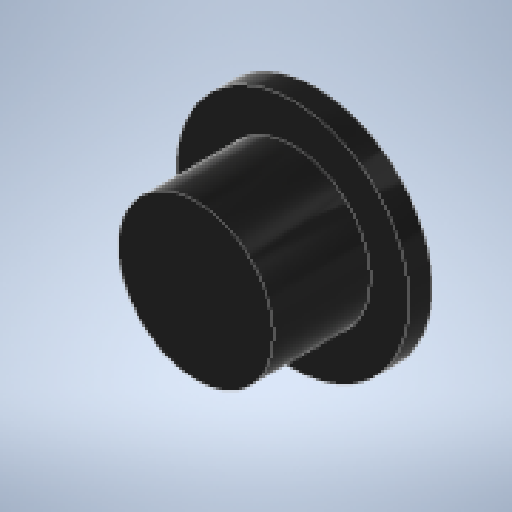
# Autodesk Inventor part: bouton
Saved by Autodesk Inventor 2024.2 (Build 282272000, 272)
## iProperties
Created: 2024-09-16
Part Number: bouton
Material: Plastique ABS
Document SubType Name: Modeling
Designer: Sebastien
Density: 1.06 g/cm^3
Appearance: Lisse - Noir
Author: Sebastien
Autodesk Inventor part; units mm, degrees
ref_plane "YZ Plane" through (0, 0, 0) normal (1, 0, 0) x (0, 1, 0)
ref_plane "XZ Plane" through (0, 0, 0) normal (0, 1, 0) x (-1, 0, 0)
ref_plane "XY Plane" through (0, 0, 0) normal (0, 0, 1) x (1, 0, 0)
sketch "Esquisse1" plane through (0, 0, 0) normal (1, 0, 0) x (0, 1, 0)
  line L0 (0, 0) -> (0, -3.1)
  line L1 (0, -3.1) -> (3, -3.1)
  line L2 (3, -3.1) -> (3, -2.5)
  line L3 (3, -2.5) -> (2, -2.5)
  line L4 (2, -2.5) -> (2, 0)
  line L5 (2, 0) -> (0, 0)
  dimension "d0" = 4
  dimension "d1" = 2.5
  dimension "d2" = 0.6
  dimension "d3" = 6
  constraints: 12 end point, 5 perpendicular, 1 vertical
  measures "d0" diameter of L4 L0
  measures "d1" distance of L3.end L4.end
  measures "d2" distance of L1.end L2.end
  measures "d3" diameter of L2 L0
revolve "Révolution1" add sketch "Esquisse1" angle 360 about axis through (0, 0, 0) along (0, 0, -1)
